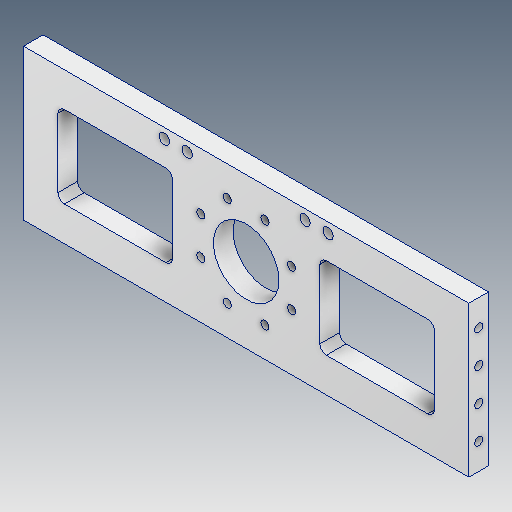
# Autodesk Inventor part: 조인트3힌지윗판_6T
Saved by Autodesk Inventor 2020.5 (Build 245400000, 400)
## iProperties
Created: 2022-01-24
Part Number: 조인트3힌지윗판_6T
Material: 알루미늄 6061
Document SubType Name: Modeling
Designer: BAEK
Density: 2.7 g/cm^3
Appearance: 알루미늄 - 평지
Mass: 66.2256 g
Surface Area: 132.096 cm^2
Volume: 24.528 cm^3
Author: BAEK
Autodesk Inventor part; units mm, degrees
ref_plane "YZ Plane" through (0, 0, 0) normal (1, 0, 0) x (0, 1, 0)
ref_plane "XZ Plane" through (0, 0, 0) normal (0, 1, 0) x (-1, 0, 0)
ref_plane "XY Plane" through (0, 0, 0) normal (0, 0, 1) x (1, 0, 0)
sketch "스케치1" plane through (0, 0, 0) normal (0, 0, 1) x (1, 0, 0)
  line L0 (0, 0) -> (0, 46)
  line L1 (0, 46) -> (136, 46)
  line L2 (136, 46) -> (136, 0)
  line L3 (136, 0) -> (0, 0)
  dimension "d0" = 46
  dimension "d1" = 136
  constraints: 8 end point, 2 perpendicular, 1 horizontal, 1 vertical
  measures "d0" distance of L0.start L0.end
  measures "d1" distance of L0.end L1.end
extrude "돌출1" add sketch "스케치1" along normal blind 6
sketch "스케치2" plane through (0, 0, 6) normal (0, 0, 1) x (1, 0, 0)
  line L0 (0, 46) -> (0, 0) projected
  line L1 (0, 23) -> (136, 23) construction
  line L2 (136, 0) -> (136, 46) projected
  line L3 (136, 46) -> (0, 46) projected
  line L4 (68, 46) -> (68, 0) construction
  line L5 (0, 0) -> (136, 0) projected
  circle A0 centre (68, 23) radius 14
  line L6 (68, 23) -> (62.2597, 36.8582)
  line L7 (68.3516, 23) -> (83.3516, 23) construction
  circle A1 centre (62.2597, 36.8582) radius 1.25
  circle A2 centre (54.1418, 28.7403) radius 1.25
  circle A3 centre (54.1418, 17.2597) radius 1.25
  circle A4 centre (62.2597, 9.1418) radius 1.25
  circle A5 centre (73.7403, 9.1418) radius 1.25
  circle A6 centre (81.8582, 17.2597) radius 1.25
  circle A7 centre (81.8582, 28.7403) radius 1.25
  circle A8 centre (73.7403, 36.8582) radius 1.25
  circle A9 centre (68, 23) radius 0.245
  dimension "d30" = 28
  dimension "d31" = 15
  dimension "d32" = 112.5
  dimension "d33" = 2.5
  dimension "d34" = 360
  constraints: 10 centre point, 8 end point, 5 midpoint, 2 coincident, 1 equal length, 1 horizontal, 1 other
  measures "d30" diameter of A0
  measures "d31" distance of L6.start L6.end
  measures "d32" angle of L7 L6
  measures "d33" diameter of A1
extrude "돌출2" cut sketch "스케치2" against normal blind 6 contours A7 A0 | A0 A7 | A6 A0 | A0 A6 | A8 A0 | A0 A8 | A5 A0 | A0 A5 | A1 L6 A0 | A0 A1 | A4 A0 | A0 A4 | L6 A1 A0 | A3 A0 | A0 A3 | A2 A0 | A0 A2
sketch "스케치3" plane through (0, 0, 6) normal (0, 0, 1) x (1, 0, 0)
  line L0 (0, 46) -> (0, 0) projected
  line L1 (0, 23) -> (136, 23) construction
  line L2 (136, 0) -> (136, 46) projected
  line L3 (136, 46) -> (0, 46) projected
  line L4 (68, 46) -> (68, 0) construction
  line L5 (0, 0) -> (136, 0) projected
  circle A0 centre (68, 23) radius 10
  dimension "d13" = 20
  constraints: 5 midpoint, 4 end point, 1 centre point
  measures "d13" diameter of A0
extrude "돌출3" cut sketch "스케치3" against normal blind 6 contours A0
sketch "스케치4" plane through (136, 0, 0) normal (1, 0, 0) x (0, 0, -1)
  line L0 (0, 0) -> (-6, 0) projected
  line L1 (-3, 0) -> (-3, 46) construction
  line L2 (0, 46) -> (-6, 46) projected
  circle A0 centre (-3, 38) radius 1.25
  circle A1 centre (-3, 28) radius 1.25
  circle A2 centre (-3, 18) radius 1.25
  circle A3 centre (-3, 8) radius 1.25
  dimension "d16" = 2.5
  dimension "d17" = 2.5
  dimension "d18" = 2.5
  dimension "d19" = 2.5
  dimension "d20" = 10
  dimension "d21" = 10
  dimension "d22" = 10
  dimension "d23" = 8
  constraints: 4 centre point, 4 point on line, 2 end point, 2 midpoint
  measures "d16" diameter of A0
  measures "d17" diameter of A1
  measures "d18" diameter of A2
  measures "d19" diameter of A3
  measures "d20" distance of A2.centre A3.centre
  measures "d21" distance of A1.centre A2.centre
  measures "d22" distance of A1.centre A0.centre
  measures "d23" distance of L1.end A0.centre
extrude "돌출4" cut sketch "스케치4" against normal blind 6
sketch "스케치5" plane through (0, 0, 0) normal (-1, 0, 0) x (0, 0, 1)
  line L0 (0, 46) -> (6, 46) projected
  line L1 (0, 0) -> (6, 0) projected
  circle A0 centre (3, 38) radius 1.25 projected
  circle A1 centre (3, 28) radius 1.25 projected
  circle A2 centre (3, 18) radius 1.25 projected
  circle A3 centre (3, 8) radius 1.25 projected
extrude "돌출5" cut sketch "스케치5" against normal blind 6
sketch "스케치6" plane through (0, 0, 6) normal (0, 0, 1) x (1, 0, 0)
  circle A0 centre (68, 23) radius 10 projected
  circle A1 centre (81.8582, 17.2597) radius 1.25 projected
  circle A2 centre (54.1418, 28.7403) radius 1.25 projected
  circle A3 centre (54.1418, 17.2597) radius 1.25 projected
  circle A4 centre (73.7403, 36.8582) radius 1.25 projected
  circle A5 centre (73.7403, 9.1418) radius 1.25 projected
  circle A6 centre (62.2597, 36.8582) radius 1.25 projected
  circle A7 centre (62.2597, 9.1418) radius 1.25 projected
  circle A8 centre (81.8582, 28.7403) radius 1.25 projected
  line L0 (136, 46) -> (0, 46) projected
  line L1 (0, 46) -> (0, 0) projected
  line L2 (0, 0) -> (136, 0) projected
  line L3 (136, 0) -> (136, 46) projected
  line L4 (12.5, 35.5) -> (43.5, 35.5)
  line L5 (45.5, 33.5) -> (45.5, 12.5)
  line L6 (43.5, 10.5) -> (12.5, 10.5)
  line L7 (10.5, 12.5) -> (10.5, 33.5)
  line L8 (136, 46) -> (0, 46) projected
  line L9 (68, 46) -> (68, 0) construction
  line L10 (0, 0) -> (136, 0) projected
  line L11 (123.5, 35.5) -> (92.5, 35.5)
  line L12 (90.5, 33.5) -> (90.5, 12.5)
  line L13 (92.5, 10.5) -> (123.5, 10.5)
  line L14 (125.5, 12.5) -> (125.5, 33.5)
  arc A9 (45.5, 33.5) -> (43.5, 35.5) centre (43.5, 33.5) ccw
  arc A10 (43.5, 10.5) -> (45.5, 12.5) centre (43.5, 12.5) ccw
  arc A11 (10.5, 12.5) -> (12.5, 10.5) centre (12.5, 12.5) ccw
  arc A12 (92.5, 35.5) -> (90.5, 33.5) centre (92.5, 33.5) ccw
  arc A13 (125.5, 33.5) -> (123.5, 35.5) centre (123.5, 33.5) ccw
  arc A14 (123.5, 10.5) -> (125.5, 12.5) centre (123.5, 12.5) ccw
  arc A15 (90.5, 12.5) -> (92.5, 10.5) centre (92.5, 12.5) ccw
  arc A16 (12.5, 35.5) -> (10.5, 33.5) centre (12.5, 33.5) ccw
  point P0 (10.5, 35.5)
  point P1 (45.5, 10.5)
  point P2 (45.5, 35.5)
  point P3 (10.5, 10.5)
  point P4 (125.5, 35.5)
  point P5 (90.5, 10.5)
  point P6 (90.5, 35.5)
  point P7 (125.5, 10.5)
  dimension "d35" = 35
  dimension "d36" = 25
  dimension "d37" = 10.5
  dimension "d38" = 10.5
  dimension "d41" = 2
  dimension "d42" = 2
  constraints: 18 end point, 16 point on circle, 16 point on line, 16 tangent, 8 centre point, 6 equal radius, 4 symmetric about line, 2 midpoint, 2 parallel, 1 horizontal, 1 perpendicular
  measures "d35" distance of point (10.5, 35.5) point (45.5, 35.5)
  measures "d36" distance of point (10.5, 10.5) point (10.5, 35.5)
  measures "d37" distance between parallel lines of L2 L6
  measures "d38" distance between parallel lines of L1 L7
  measures "d41" radius of A9
  measures "d42" radius of A16
extrude "돌출6" cut sketch "스케치6" against normal blind 6 contours L4 A9 L5 A10 L6 A11 L7 A16 | A13 L14 A14 L13 A15 L12 A12 L11
sketch "스케치11" plane through (0, 0, 6) normal (0, 0, 1) x (1, 0, 0)
  line L0 (136, 46) -> (0, 46) projected
  line L1 (68, 46) -> (68, 43)
  line L2 (136, 43) -> (0, 43) construction
  circle A0 centre (50, 43) radius 1.6
  circle A1 centre (86, 43) radius 1.6
  circle A2 centre (43, 43) radius 1.6
  circle A3 centre (93, 43) radius 1.6
  point P0 (0, 0)
  dimension "d67" = 3
  dimension "d69" = 3
  dimension "d70" = 3.2
  dimension "d71" = 3.2
  dimension "d72" = 18
  dimension "d73" = 18
  dimension "d74" = 3.2
  dimension "d75" = 3.2
  dimension "d76" = 7
  dimension "d77" = 7
  constraints: 4 centre point, 4 end point, 4 point on line, 1 midpoint, 1 parallel, 1 vertical
  measures "d67" distance of L1.start L1.end
  measures "d69" distance between parallel lines of L0 L2
  measures "d70" diameter of A0
  measures "d71" diameter of A1
  measures "d72" distance of A0.centre L1.end
  measures "d73" distance of A1.centre L1.end
  measures "d74" diameter of A2
  measures "d75" diameter of A3
  measures "d76" distance of A2.centre A0.centre
  measures "d77" distance of A1.centre A3.centre
extrude "돌출8" cut sketch "스케치11" against normal blind 10
